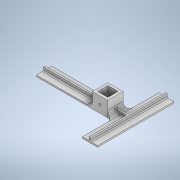
# Autodesk Inventor part: uv_stand
Saved by Autodesk Inventor 2020 (Build 240168000, 168)
## iProperties
Created: 2020-04-27
Part Number: uv_stand
Material: Generic
Document SubType Name: Modeling
Designer: Clevo
Density: 1 g/cm^3
Appearance: Default
Author: Clevo
Autodesk Inventor part; units mm, degrees
ref_plane "YZ Plane" through (0, 0, 0) normal (1, 0, 0) x (0, 1, 0)
ref_plane "XZ Plane" through (0, 0, 0) normal (0, 1, 0) x (-1, 0, 0)
ref_plane "XY Plane" through (0, 0, 0) normal (0, 0, 1) x (1, 0, 0)
sketch "Sketch1" plane through (0, 0, 0) normal (0, 1, 0) x (-1, 0, 0)
  line L0 (-15, -75) -> (15, -75)
  line L1 (15, -75) -> (15, 75)
  line L2 (15, 75) -> (-15, 75)
  line L3 (-15, 75) -> (-15, -75)
  line L4 (-15, -75) -> (15, 75) construction
  line L5 (15, -75) -> (-15, 75) construction
  line L6 (15, 15) -> (165, 15)
  line L7 (165, 15) -> (165, -15)
  line L8 (165, -15) -> (15, -15)
  line L9 (15, -15) -> (15, 15)
  point P0 (0, 0)
  point P1 (165, 0)
  point P2 (0, 0)
  point P3 (15, -15)
  dimension "d0" = 150
  dimension "d1" = 30
  dimension "d2" = 150
  dimension "d3" = 30
  constraints: 20 end point, 4 midpoint, 4 parallel, 2 horizontal, 2 perpendicular, 1 horizontal alignment, 1 point on line
  measures "d0" distance of L2.end L0.start
  measures "d1" distance of L0.start L0.end
  measures "d2" distance of L7.end L8.end
  measures "d3" distance of L6.end L7.end
extrude "Extrusion1" add sketch "Sketch1" along normal blind 3
sketch "Sketch2" plane through (0, 3, 0) normal (0, 1, 0) x (1, 0, 0)
  line L0 (-55, -15) -> (-25, -15)
  line L1 (-25, -15) -> (-25, 15)
  line L2 (-25, 15) -> (-55, 15)
  line L3 (-55, 15) -> (-55, -15)
  line L4 (-55, -15) -> (-25, 15) construction
  line L5 (-25, -15) -> (-55, 15) construction
  point P0 (0, 0)
  point P1 (-40, 0)
  dimension "d6" = 30
  dimension "d7" = 30
  dimension "d8" = 40
  constraints: 12 end point, 2 midpoint, 2 parallel, 1 horizontal, 1 perpendicular
  measures "d6" distance of L2.end L0.start
  measures "d7" distance of L1.end L2.end
  measures "d8" distance of point (0, 0) point (-40, 0)
extrude "Extrusion2" add sketch "Sketch2" along normal blind 30 from surface at -3
sketch "Sketch4" plane through (-55, 30, 15) normal (0, 1, 0) x (1, 0, 0)
  line L0 (0, 0) -> (0, 30) projected
  line L1 (30, 0) -> (0, 0) projected
  line L2 (30, 30) -> (30, 0) projected
  line L3 (0, 30) -> (30, 30) projected
  line L4 (25.125, 4.875) -> (4.875, 4.875)
  line L5 (4.875, 4.875) -> (4.875, 25.125)
  line L6 (4.875, 25.125) -> (25.125, 25.125)
  line L7 (25.125, 25.125) -> (25.125, 4.875)
  line L8 (25.125, 4.875) -> (4.875, 25.125) construction
  line L9 (4.875, 4.875) -> (25.125, 25.125) construction
  point P0 (55, 15)
  point P1 (15, 15)
  point P2 (15, 15)
  point P3 (30, 15)
  point P4 (15, 15)
  point P5 (15, 30)
  dimension "d11" = 20.25
  dimension "d12" = 20.25
  constraints: 12 end point, 6 midpoint, 2 parallel, 1 horizontal, 1 horizontal alignment, 1 perpendicular, 1 vertical alignment
  measures "d11" distance of L5.end L6.end
  measures "d12" distance of L4.end L5.end
extrude "Extrusion3" cut sketch "Sketch4" against normal through all contours L4 L5 L6 L7
fillet "Fillet1" radius 10 4 edges at (-25, 3, 0) (-15, 1.5, 15) (-15, 1.5, -15) (-55, 3, 0)
sketch "Sketch5" plane through (-55, 30, 15) normal (0, 0, 1) x (1, 0, 0)
  line L0 (30, -17) -> (30, -30) projected
  line L1 (30, 0) -> (30, -17) projected
  line L2 (30, 0) -> (0, 0) projected
  line L3 (0, -17) -> (0, 0) projected
  arc A0 (-10, -27) -> (0, -17) centre (-10, -17) ccw projected
  line L4 (-110, -27) -> (-10, -27) projected
  line L5 (-110, -30) -> (-110, -27) projected
  line L6 (-110, -30) -> (30, -30) projected
  point P0 (55, -30)
  point P1 (15, -15)
  point P2 (15, 0)
  dimension "d16" = 15
  constraints: 1 midpoint, 1 vertical alignment
  measures "d16" distance from line of L6 point (15, -15)
hole "Hole1" at (-40, 15, 15) direction (0, 0, -1) diameter 4.3 end through all clearance for "Flat Head Machine Screw" size "M4" standard "Ansi Metric M Profile"
sketch "Sketch6" plane through (0, 0, 0) normal (0, -1, 0) x (1, 0, 0)
  line L0 (-50.125, 10.125) -> (-29.875, 10.125) projected
  line L1 (-29.875, 10.125) -> (-29.875, -10.125) projected
  line L2 (-29.875, -10.125) -> (-50.125, -10.125) projected
  line L3 (-50.125, -10.125) -> (-50.125, 10.125) projected
  line L4 (-165, 15) -> (-25, 15) projected
  line L5 (-165, -15) -> (-165, 15) projected
  line L6 (-25, -15) -> (-165, -15) projected
  arc A0 (-15, -25) -> (-25, -15) centre (-25, -25) ccw projected
  line L7 (-15, -75) -> (-15, -25) projected
  line L8 (15, -75) -> (-15, -75) projected
  line L9 (15, 75) -> (15, -75) projected
  line L10 (-15, 75) -> (15, 75) projected
  line L11 (-15, 25) -> (-15, 75) projected
  arc A1 (-25, 15) -> (-15, 25) centre (-25, 25) ccw projected
  line L12 (-50.125, 10.125) -> (-50.125, -10.125) projected
  line L13 (-165, 1.5) -> (-50.125, 1.5)
  line L14 (-50.125, 1.5) -> (-50.125, -1.5)
  line L15 (-50.125, -1.5) -> (-165, -1.5)
  line L16 (-165, -1.5) -> (-165, 1.5)
  line L17 (-165, 1.5) -> (-50.125, -1.5) construction
  line L18 (-50.125, 1.5) -> (-165, -1.5) construction
  line L19 (1.5, -75) -> (-1.5, -75)
  line L20 (-1.5, -75) -> (-1.5, 75)
  line L21 (-1.5, 75) -> (1.5, 75)
  line L22 (1.5, 75) -> (1.5, -75)
  line L23 (1.5, -75) -> (-1.5, 75) construction
  line L24 (-1.5, -75) -> (1.5, 75) construction
  line L25 (-28.5, 1.5) -> (-1.5, 1.5)
  line L26 (-1.5, 1.5) -> (-1.5, -1.5)
  line L27 (-1.5, -1.5) -> (-28.5, -1.5)
  line L28 (-28.5, -1.5) -> (-28.5, 1.5)
  line L29 (-15, -25) -> (-15, 25) projected
  line L30 (-28.5, 1.5) -> (-1.5, -1.5) construction
  line L31 (-1.5, 1.5) -> (-28.5, -1.5) construction
  line L32 (-165, -15) -> (-165, 15) projected
  line L33 (-15, 75) -> (15, 75) projected
  point P0 (0, 0)
  point P1 (-107.5625, 0)
  point P2 (-15, 0)
  point P3 (-107.5625, 0)
  point P4 (-50.125, 0)
  point P5 (-1.5, -1.5)
  point P6 (-1.5, 75)
  point P7 (-1.5, 1.5)
  dimension "d24" = 3
  dimension "d25" = 3
  dimension "d26" = 3
  constraints: 36 end point, 9 midpoint, 6 parallel, 3 collinear, 3 horizontal, 3 perpendicular, 1 horizontal alignment, 1 point on line
  measures "d24" distance between parallel lines of L20 L22
  measures "d25" distance between parallel lines of L27 L25
  measures "d26" distance between parallel lines of L13 L15
extrude "Extrusion4" add sketch "Sketch6" against normal blind 10 contours L3 L15 L5 L13 | L29 L27 L28 L25 | L25 L20 L27 L29 | L10 L22 L8 L20
fillet "Fillet2" radius 2 11 edges at (-115, 3, 1.5) (-59.0839, 4.9377, 1.5) (-59.0839, 4.9377, -1.5) (-115, 3, -1.5) (-20.9161, 4.9377, 1.5) (-8.25, 3, 1.5) (-1.5, 3, 38.25) (1.5, 3, 0) (-1.5, 3, -38.25) (-20.9161, 4.9377, -1.5) (-8.25, 3, -1.5)
equation "\"d2\" = d0"
equation "\"d3\" = d1"
equation "\"d7\" = d6"
body "Solid1"
